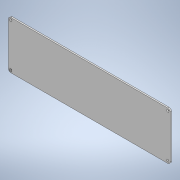
# Autodesk Inventor part: Acrylic Front Plate
Saved by Autodesk Inventor 2020 (Build 240168000, 168)
## iProperties
Created: 2021-04-14
Part Number: Acrylic Front Plate
Material: Generic
Document SubType Name: Modeling
Designer: user
Density: 1 g/cm^3
Appearance: Default
Author: user
Autodesk Inventor part; units mm, degrees
ref_plane "YZ Plane" through (0, 0, 0) normal (1, 0, 0) x (0, 1, 0)
ref_plane "XZ Plane" through (0, 0, 0) normal (0, 1, 0) x (-1, 0, 0)
ref_plane "XY Plane" through (0, 0, 0) normal (0, 0, 1) x (1, 0, 0)
sketch "Sketch1" plane through (0, 0, 0) normal (0, 0, 1) x (1, 0, 0)
  line L0 (0, 0) -> (323, 0)
  line L1 (323, 0) -> (323, 83)
  line L2 (323, 83) -> (0, 83)
  line L3 (0, 83) -> (0, 0)
  line L4 (-9, 92) -> (332, 92)
  line L5 (332, 92) -> (332, -9)
  line L6 (332, -9) -> (-9, -9)
  line L7 (-9, -9) -> (-9, 92)
  dimension "d0" = 323
  dimension "d1" = 83
  dimension "d2" = 9
  constraints: 16 end point, 4 parallel, 2 perpendicular, 1 horizontal, 3 other
  measures "d0" distance of L2.end L1.end
  measures "d1" distance of L2.end L0.start
  measures "d2" distance between parallel lines of L2 L4
extrude "Extrusion1" add sketch "Sketch1" along normal blind 3 contours L3 L2 L1 L0 | L4 L5 L6 L7
sketch "Sketch2" plane through (0, 0, 3) normal (0, 0, 1) x (1, 0, 0)
  circle A0 centre (-4, 87) radius 2.6
  line L0 (332, 92) -> (-9, 92) projected
  line L1 (-9, 92) -> (-9, -9) projected
  line L2 (0, 0) -> (323, 0)
  line L3 (323, 0) -> (323, 83)
  line L4 (323, 83) -> (0, 83)
  line L5 (0, 83) -> (0, 0)
  line L6 (-9, -9) -> (332, -9) projected
  line L7 (332, -9) -> (332, 92) projected
  circle A1 centre (-4, 87) radius 3.5
  circle A2 centre (-4, -4) radius 2.6
  circle A3 centre (327, -4) radius 2.5
  circle A4 centre (327, 87) radius 2.5
  point P0 (0, 0)
  dimension "d6" = 5.2
  dimension "d9" = 9
  dimension "d10" = 9
  dimension "d11" = 9
  dimension "d12" = 9
  dimension "d15" = 7
  dimension "d16" = 5
  dimension "d17" = 5
  dimension "d18" = 5.2
  dimension "d19" = 5
  dimension "d20" = 5
  dimension "d21" = 5
  dimension "d22" = 5
  dimension "d23" = 5
  dimension "d24" = 5
  dimension "d25" = 5
  dimension "d26" = 5
  constraints: 8 end point, 5 centre point, 2 parallel, 1 coincident, 1 horizontal, 1 perpendicular
  measures "d6" diameter of A0
  measures "d9" distance between parallel lines of L4 L0
  measures "d10" distance between parallel lines of L6 L2
  measures "d11" distance between parallel lines of L5 L1
  measures "d12" distance between parallel lines of L7 L3
  measures "d15" diameter of A1
  measures "d16" distance from line of L0 A0.centre
  measures "d17" distance from line of L1 A0.centre
  measures "d18" diameter of A2
  measures "d19" distance from line of L1 A2.centre
  measures "d20" distance from line of L6 A2.centre
  measures "d21" diameter of A3
  measures "d22" distance from line of L7 A3.centre
  measures "d23" distance from line of L6 A3.centre
  measures "d24" diameter of A4
  measures "d25" distance from line of A4.centre L0
  measures "d26" distance from line of L7 A4.centre
extrude "Extrusion2" cut sketch "Sketch2" against normal blind 3 contours A0 | A2 | A3 | A4
fillet "Fillet2" radius 5 4 edges at (332, 92, 1.5) (332, -9, 1.5) (-9, 92, 1.5) (-9, -9, 1.5)
body "Solid1"
